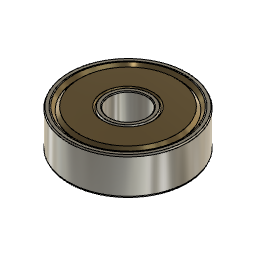
ANEMOMETR SESTAVA v3 (Autodesk Fusion 360 archive; units mm, degrees)
design "Ložisko"
Autodesk Fusion 360 part; units mm, degrees
note: some values were not read from the file. Chosen so that the rebuilt part matches the saved one: which bodies a step acts on; which face or edge a step refers to. Set by a fixed rule: which sketch regions a step uses.
sketch "Sketch1" plane through (0, 0, 0) normal (0, 0, 1) x (1, 0, 0)
  circle A0 centre (50, 25) radius 8
  circle A1 centre (50, 25) radius 2.5
  dimension "d1" = 16
  dimension "d2" = 5
  constraint concentric A0 A1
  measures "d1" diameter of A0
  measures "d2" diameter of A1
extrude "Extrude1" add sketch "Sketch1" along normal blind 5 makes body 1
sketch "Sketch2" plane through (0, 0, 5) normal (0, 0, 1) x (-1, 0, 0)
  circle A0 centre (-50, -25) radius 2.5
  circle A1 centre (-50, -25) radius 8
  circle A2 centre (-50, -25) radius 3
  circle A3 centre (-50, -25) radius 3.15
  circle A4 centre (-50, -25) radius 7.5
  circle A5 centre (-50, -25) radius 7.35
  dimension "d5" = 6
  dimension "d6" = 6.3
  dimension "d7" = 15
  dimension "d8" = 14.7
  constraint concentric A0 A2
  constraint concentric A0 A3
  constraint concentric A0 A4
  constraint concentric A3 A5
  measures "d5" diameter of A2
  measures "d6" diameter of A3
  measures "d7" diameter of A4
  measures "d8" diameter of A5
extrude "Extrude2" cut sketch "Sketch2" against normal blind 9 contours A3 | A4 bodies 1 makes body 2 at (57.9901, 24.6012, 3.3333) makes body 3 at (47.0149, 25.2987, 3.3333)
sketch "Sketch3" plane through (0, 0, 5) normal (0, 0, 1) x (-1, 0, 0)
  circle A0 centre (-50, -25) radius 3.15
  circle A1 centre (-50, -25) radius 7.35
  circle A2 centre (-50, -25) radius 6.5
  dimension "d11" = 13
  constraint concentric A0 A2
  measures "d11" diameter of A2
extrude "Extrude3" cut sketch "Sketch3" against normal blind 1 draft -45 contours A1 bodies 1
sketch "Sketch4" plane through (0, 0, 0) normal (0, 0, -1) x (1, 0, 0)
  circle A0 centre (50, -25) radius 3.15
  circle A1 centre (50, -25) radius 7.35
  circle A2 centre (50, -25) radius 6.5
  dimension "d14" = 13
  constraint concentric A0 A2
  measures "d14" diameter of A2
extrude "Extrude4" cut sketch "Sketch4" against normal blind 1.5 draft -45 contours A1 bodies 1
chamfer "Chamfer1" distance 0.2 angle 45 1 edges at (52.9368, 23.8609, 5) on bodies 1
chamfer "Chamfer2" distance 0.2 angle 45 1 edges at (52.9368, 26.1391, 0) on bodies 1
chamfer "Chamfer3" distance 0.1 angle 65 1 edges at (42.5414, 22.1071, 5) measured on face at (57.7756, 24.2299, 5) on bodies 2
chamfer "Chamfer4" distance 0.2 angle 25 1 edges at (42.5414, 22.1071, 0) measured on face at (57.9901, 24.6012, 3.1904) on bodies 2
chamfer "Chamfer5" distance 0.1 angle 45 2 edges at (47.6692, 25.904, 0) (47.6692, 25.904, 5) measured on face at (52.4969, 24.8754, 3.3333) measured on face at (47.1871, 25.2732, 5) on bodies 3

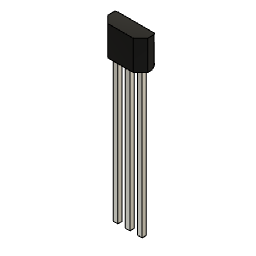
design "A3144 hall"
Autodesk Fusion 360 part; units mm, degrees
sketch "Sketch1" plane through (0, 0, 0) normal (0, 0, 1) x (1, 0, 0)
  line L0 (50, 25) -> (54.17, 25)
  line L1 (54.17, 25) -> (54.17, 24.18)
  line L2 (53.42, 23.43) -> (50.75, 23.43)
  line L3 (50, 24.18) -> (50, 25)
  line L4 (50, 24.25) -> (54.17, 24.25)
  line L5 (50, 24.18) -> (50.75, 23.43)
  line L6 (53.42, 23.43) -> (54.17, 24.18)
  point P0 (50, 25)
  point P1 (54.17, 25)
  point P2 (54.17, 23.43)
  point P3 (50, 23.43)
  dimension "d1" = 4.17
  dimension "d2" = 1.57
  dimension "d3" = 0.75
  dimension "d4" = 0.75
  dimension "d5" = 0.75
  dimension "d6" = 0.75
  constraint horizontal L0
  constraint vertical L1
  constraint horizontal L2
  constraint vertical L3
  constraint coincident L3 L4.start
  constraint coincident P3 L3
  constraint coincident P3 L2
  constraint coincident L1 L4.end
  constraint coincident P2 L2
  constraint coincident P2 L1
  constraint coincident P0 L0
  constraint coincident P0 L3
  constraint coincident P1 L0
  constraint coincident P1 L1
  constraint coincident P0 L0.start
  constraint coincident P1 L0.end
  measures "d1" distance of P0 L0.end
  measures "d2" distance of P0 P3
  measures "d3" distance of P3 L3.start
  measures "d4" distance of P3 L2.end
  measures "d5" distance of P2 L2.start
  measures "d6" distance of P2 L1.end
extrude "Extrude1" add sketch "Sketch1" along normal blind 3.1 makes body 1
sketch "Sketch2" plane through (0, 0, 0) normal (0, 0, -1) x (1, 0, 0)
  line L0 (54.17, -24.18) -> (53.42, -23.43)
  line L1 (53.42, -23.43) -> (50.75, -23.43)
  line L2 (50.75, -23.43) -> (50, -24.18)
  line L3 (50, -24.18) -> (50, -25)
  line L4 (50, -25) -> (54.17, -25)
  line L5 (54.17, -25) -> (54.17, -24.18)
  line L6 (54.17, -24.18) -> (50, -24.18)
  line L7 (52.085, -23.43) -> (52.085, -25)
  line L8 (51.845, -24.62) -> (52.325, -24.62)
  line L9 (52.325, -24.62) -> (52.325, -24.18)
  line L10 (52.325, -24.18) -> (51.845, -24.18)
  line L11 (51.845, -24.18) -> (51.845, -24.62)
  line L12 (53.595, -24.18) -> (53.115, -24.18)
  line L13 (53.115, -24.18) -> (53.115, -24.62)
  line L14 (53.595, -24.62) -> (53.595, -24.18)
  line L15 (53.115, -24.62) -> (53.595, -24.62)
  line L16 (51.055, -24.18) -> (50.575, -24.18)
  line L17 (50.575, -24.18) -> (50.575, -24.62)
  line L18 (50.575, -24.62) -> (51.055, -24.62)
  line L19 (51.055, -24.62) -> (51.055, -24.18)
  dimension "d13" = 0.48
  dimension "d14" = 0.44
  dimension "d16" = 0.48
  dimension "d17" = 0.44
  dimension "d18" = 0.48
  dimension "d19" = 0.44
  constraint coincident L0.start L5.end
  constraint coincident L2.end L3.start
  constraint midpoint L1 L7.start
  constraint midpoint L4 L7.end
  constraint horizontal L8
  constraint vertical L9
  constraint horizontal L10
  constraint vertical L11
  constraint horizontal L15
  constraint vertical L14
  constraint horizontal L12
  constraint vertical L13
  constraint horizontal L18
  constraint vertical L19
  constraint horizontal L16
  constraint vertical L17
  measures "d13" distance of L8.start L8.end
  measures "d14" distance of L8.start L10.end
  measures "d16" distance of L13.end L14.start
  measures "d17" distance of L13.end L12.end
  measures "d18" distance of L17.end L18.end
  measures "d19" distance of L17.end L16.end
extrude "Extrude2" add sketch "Sketch2" along normal blind 15.24 separate body contours L6 L12 L13 L14 L15 | L6 L7 L8 L10 L11 | L6 L7 L8 L9 L10 | L6 L16 L17 L18 L19 makes body 2 at (50.735, 24.62, -5.08) makes body 3 at (52.165, 24.18, -5.08) makes body 4 at (53.435, 24.18, -5.08)
chamfer "Chamfer1" distance 0.38 angle 45 1 edges at (52.085, 25, 0) on bodies 1
fillet "Fillet1" radius 0.15 2 edges at (54.17, 25, 1.74) (50, 25, 1.74) on bodies 1
equation "d4 = d3"
equation "d6 = d5"

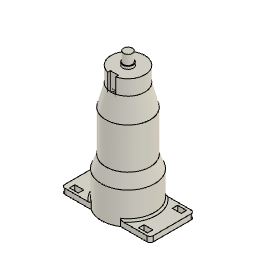
design "Anemometr_spodnidil"
Autodesk Fusion 360 part; units mm, degrees
sketch "Sketch1" plane through (0, 0, 0) normal (0, 0, 1) x (1, 0, 0)
  line L0 (0, 0) -> (7, 0)
  line L1 (7, 0) -> (7, 7)
  line L2 (7, 7) -> (0, 7)
  line L3 (0, 7) -> (0, 0)
  line L4 (7, 7) -> (-7, 7)
  line L5 (-7, 7) -> (-7, -7)
  line L6 (-7, -7) -> (7, -7)
  line L7 (7, -7) -> (7, 7)
  line L8 (0, 0) -> (25, 0)
  line L9 (25, 0) -> (25, 12.5)
  line L10 (25, 12.5) -> (0, 12.5)
  line L11 (0, 12.5) -> (0, 0)
  line L12 (25, 12.5) -> (-25, 12.5)
  line L13 (-25, 12.5) -> (-25, -12.5)
  line L14 (-25, -12.5) -> (25, -12.5)
  line L15 (25, -12.5) -> (25, 12.5)
  dimension "d1" = 7
  dimension "d2" = 7
  dimension "d3" = 14
  dimension "d4" = 14
  dimension "d5" = 25
  dimension "d6" = 12.5
  dimension "d7" = 50
  dimension "d8" = 25
  constraint horizontal L0
  constraint vertical L1
  constraint horizontal L2
  constraint vertical L3
  constraint coincident L0.start L3.end
  constraint horizontal L4
  constraint vertical L5
  constraint horizontal L6
  constraint vertical L7
  constraint horizontal L8
  constraint vertical L9
  constraint horizontal L10
  constraint vertical L11
  constraint horizontal L12
  constraint vertical L13
  constraint horizontal L14
  constraint vertical L15
  measures "d1" distance of L0.start L0.end
  measures "d2" distance of L0.start L2.end
  measures "d3" distance of L1.end L4.end
  measures "d4" distance of L1.end L6.end
  measures "d5" distance of L0.start L8.end
  measures "d6" distance of L0.start L10.end
  measures "d7" distance of L9.end L12.end
  measures "d8" distance of L9.end L14.end
extrude "Extrude1" add sketch "Sketch1" along normal blind 3 makes body 1
sketch "Sketch2" plane through (0, 0, 3) normal (0, 0, 1) x (-1, 0, 0)
  line L0 (-25, 12.5) -> (-25, -12.5)
  line L1 (-25, -12.5) -> (25, -12.5)
  line L2 (25, -12.5) -> (25, 12.5)
  line L3 (25, 12.5) -> (-25, 12.5)
  circle A0 centre (0, 0) radius 15
  circle A1 centre (0, 0) radius 13
  dimension "d11" = 30
  dimension "d16" = 26
  constraint coincident A0.centre A1.centre
  constraint concentric A0 A1
  measures "d11" diameter of A0
  measures "d16" diameter of A1
extrude "Extrude2" add sketch "Sketch2" against normal blind 3 contours L3 A0 A1 | L1 L3 A0 A1 | L1 A0 A1 | L3 A1 | L1 L3 A1 | L1 L3 A0 A1 | L1 A1 bodies 1
extrude "Extrude4" cut sketch "Sketch2" against normal blind 22 contours L3 A1 | L1 A1 bodies 1
extrude "Extrude5" cut 1 faces at (1.1902, 12.5, 2) along direction (0, -1, 0) blind 2 on bodies 1 bodies 1
extrude "Extrude6" cut 1 faces at (-1.1902, -12.5, 2) along direction (0, 1, 0) blind 2 on bodies 1 bodies 1
sketch "Sketch4" plane through (0, 0, 0) normal (0, 1, 0) x (1, 0, 0)
  line L0 (15, -3) -> (15, -18)
  line L1 (13, -3) -> (13, -18)
  line L2 (13, -3) -> (15, -3)
  line L3 (0, 0) -> (0, -25)
  line L4 (12.5, -25) -> (15, -18)
  line L5 (13, -18) -> (10.5, -24.9905)
  line L6 (12.5, -25) -> (12.5, -48)
  line L7 (10.5, -24.9905) -> (10.5, -47.9905)
  line L8 (0, -25) -> (0, -60)
  line L9 (9.5, -60) -> (12.5, -48)
  line L10 (9.5, -60) -> (7.5, -60)
  line L11 (7.5, -60) -> (10.5, -47.9905)
  dimension "d30" = 15
  dimension "d31" = 15
  dimension "d32" = 13
  dimension "d33" = 2
  dimension "d34" = 25
  dimension "d35" = 12.5
  dimension "d36" = 25
  dimension "d37" = 2
  dimension "d38" = 23
  dimension "d39" = 2
  dimension "d43" = 9.5
  dimension "d44" = 2
  constraint perpendicular L0 L2
  constraint coincident L3.start origin
  constraint vertical L3
  constraint vertical L6
  constraint parallel L6 L7
  constraint parallel L3 L8
  constraint horizontal L10
  measures "d30" distance of L0.start L0.end
  measures "d31" distance of L1.start L1.end
  measures "d32" horizontal distance of L3.start L1.start
  measures "d33" distance of L0.start L1.start
  measures "d34" distance of L3.start L3.end
  measures "d35" distance of L3.end L4.start
  measures "d36" vertical distance of L3.start L4.start
  measures "d37" distance of L4.start L5.end
  measures "d38" distance of L5.end L7.end
  measures "d39" distance of L6.end L7.end
  measures "d43" distance of L8.end L9.start
  measures "d44" distance of L9.start L10.end
revolve "Revolve1" add sketch "Sketch4" angle 360 about axis through (0, 0, 0) along (0, 0, 1) bodies 1
extrude "Extrude8" cut sketch "Sketch2" against normal blind 20 contours L1 L3 A1 bodies 1
fillet "Fillet1" radius 1 3 edges at (13.2169, -7.0932, 3) (-15, 0, 3) (13.2169, 7.0932, 3) on bodies 1
extrude "Extrude9" add 1 faces at (8.77, -0.8446, 60) along direction (0, 0, 1) blind 8.5 on bodies 1 bodies 1
sketch "Sketch5" plane through (0, 0, 68.5) normal (0, 0, 1) x (-1, 0, 0)
  circle A0 centre (0, 0) radius 9.5
  circle A1 centre (0, 0) radius 7.5
  circle A2 centre (0, 0) radius 3
  dimension "d51" = 6
  constraint coincident A0.centre A1.centre
  measures "d51" diameter of A2
extrude "Extrude10" add sketch "Sketch5" along normal blind 1.5 separate body contours A2 makes body 2
sketch "Sketch6" plane through (0, 0, 70) normal (0, 0, 1) x (-1, 0, 0)
  circle A0 centre (0, 0) radius 3
  circle A1 centre (0, 0) radius 2.535
  dimension "d54" = 5.07
  constraint coincident A0.centre A1.centre
  measures "d54" diameter of A1
extrude "Extrude11" add sketch "Sketch6" along normal blind 5.5 contours A1 bodies 2
sketch "Sketch7" plane through (0, 0, 68.5) normal (0, 0, 1) x (-1, 0, 0)
  circle A0 centre (0, 0) radius 9.5
  circle A1 centre (0, 0) radius 7.5
  line L0 (0, 0) -> (0, 9.5)
  line L1 (0, 7.7) -> (-2.25, 7.7)
  line L2 (-2.25, 7.7) -> (2.25, 7.7)
  line L3 (2.25, 7.7) -> (2.25, 9.5)
  line L4 (2.25, 9.5) -> (-2.25, 9.5)
  line L5 (-2.25, 9.5) -> (-2.25, 7.7)
  dimension "d57" = 2.25
  dimension "d58" = 1.8
  dimension "d59" = 4.5
  dimension "d60" = 1.8
  constraint coincident A0.centre A1.centre
  constraint coincident A0 L0.end
  constraint vertical L0
  constraint coincident L0 L1.start
  constraint perpendicular L0 L1
  constraint horizontal L2
  constraint vertical L3
  constraint horizontal L4
  constraint vertical L5
  measures "d57" distance of L1.start L1.end
  measures "d58" distance of L0.end L1.start
  measures "d59" distance of L1.end L2.end
  measures "d60" distance of L1.end L4.end
extrude "Extrude12" cut sketch "Sketch7" against normal blind 16 contours A0 L0 L2 L3 | A0 L0 L1 L2 L5 bodies 1
sketch "Sketch8" plane through (0, 0, 0) normal (1, 0, 0) x (0, 1, 0)
  line L0 (9.5, 60) -> (7.5, 60)
  line L1 (7.5, 60) -> (7.5, 68.5)
  line L2 (7.5, 68.5) -> (0, 68.5)
  line L3 (7.5, 60) -> (0, 68.5)
  dimension "d63" = 2
  dimension "d64" = 8.5
  dimension "d65" = 7.5
  constraint horizontal L0
  constraint perpendicular L0 L1
  constraint perpendicular L1 L2
  measures "d63" distance of L0.start L0.end
  measures "d64" distance of L0.end L1.end
  measures "d65" distance of L1.end L2.end
revolve "Revolve2" add sketch "Sketch8" angle 360 about axis through (0, 0, 60) along (0, 0, -1) bodies 2 1
sketch "Sketch9" plane through (0, 0, 3) normal (0, 0, 1) x (-1, 0, 0)
  arc A0 (9.9875, -12.5) -> (9.9875, 12.5) centre (0, 0) ccw
  line L0 (9.9875, -12.5) -> (25, -12.5)
  line L1 (25, -12.5) -> (25, 12.5)
  line L2 (25, 12.5) -> (9.9875, 12.5)
  line L3 (22, -11) -> (17, -11)
  line L4 (17, -11) -> (17, -8)
  line L5 (17, -8) -> (22, -8)
  line L6 (22, -8) -> (22, -11)
  line L7 (0, 0) -> (25, 0)
  line L8 (22, 8) -> (22, 11)
  line L9 (22, 11) -> (17, 11)
  line L10 (17, 11) -> (17, 8)
  line L11 (17, 8) -> (22, 8)
  line L12 (0, 0) -> (0, -17)
  line L13 (-22, -8) -> (-22, -11)
  line L14 (-17, -11) -> (-17, -8)
  line L15 (-17, -8) -> (-22, -8)
  line L16 (-22, -11) -> (-17, -11)
  line L17 (-17, 11) -> (-17, 8)
  line L18 (-17, 8) -> (-22, 8)
  line L19 (-22, 11) -> (-17, 11)
  line L20 (-22, 8) -> (-22, 11)
  dimension "d68" = 5
  dimension "d69" = 3
  dimension "d70" = 8
  constraint horizontal L3
  constraint vertical L4
  constraint horizontal L5
  constraint vertical L6
  constraint coincident A0.centre L7.start
  constraint midpoint L1 L7.end
  constraint symmetric L3.start L7 L8.end
  constraint symmetric L3.end L7 L9.end
  constraint symmetric L4.end L7 L10.end
  constraint symmetric L5.end L7 L8.start
  constraint perpendicular L7 L12
  constraint symmetric L3.start L12 L13.end
  constraint symmetric L3.end L12 L14.start
  constraint symmetric L4.end L12 L14.end
  constraint symmetric L5.end L12 L13.start
  constraint symmetric L8.start L12 L18.end
  constraint symmetric L10.end L12 L17.end
  constraint symmetric L8.end L12 L19.start
  constraint symmetric L9.end L12 L17.start
  measures "d68" distance of L3.start L3.end
  measures "d69" distance of L3.start L5.end
  measures "d70" distance of L5.end L7
extrude "Extrude13" cut sketch "Sketch9" against normal blind 11 contours L3 L4 L5 L6 | L8 L9 L10 L11 | L13 L14 L15 L16 | L17 L18 L19 L20 bodies 2
fillet "Fillet2" radius 1.75 4 edges at (-25, -12.5, 1.5) (25, -12.5, 1.5) (25, 12.5, 1.5) (-25, 12.5, 1.5) on bodies 2
equation "d6 = ( 25 / 2 ) * 1 mm"
equation "d35 = ( 25 / 2 ) * 1 mm"
equation "d43 = ( 19 / 2 ) * 1 mm"
equation "d57 = ( 4.5 / 2 ) * 1 mm"
